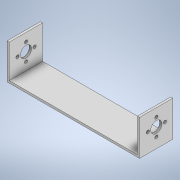
# Autodesk Inventor part: Rotate Brace
Saved by Autodesk Inventor 2020 (Build 240168000, 168)
## iProperties
Created: 2020-01-19
Part Number: Rotate Brace
Material: Generic
Document SubType Name: Modeling
Designer: tdmp4
Density: 1 g/cm^3
Appearance: Default
Author: tdmp4
Autodesk Inventor part; units mm, degrees
ref_plane "YZ Plane" through (0, 0, 0) normal (1, 0, 0) x (0, 1, 0)
ref_plane "XZ Plane" through (0, 0, 0) normal (0, 1, 0) x (-1, 0, 0)
ref_plane "XY Plane" through (0, 0, 0) normal (0, 0, 1) x (1, 0, 0)
sketch "Sketch1" plane through (0, 0, 0) normal (0, 1, 0) x (-1, 0, 0)
  line L0 (0, 0) -> (151.4602, 0)
  line L1 (151.4602, 0) -> (151.4602, -38.1)
  line L2 (151.4602, -38.1) -> (0, -38.1)
  line L3 (0, -38.1) -> (0, 0)
  dimension "d0" = 151.4602
  dimension "d1" = 38.1
  constraints: 8 end point, 2 parallel, 1 horizontal, 1 perpendicular
  measures "d0" distance of L1.end L2.end
  measures "d1" distance of L2.end L0.start
extrude "Extrusion1" add sketch "Sketch1" along normal blind 2.54
sketch "Sketch3" plane through (0, 0, 0) normal (1, 0, 0) x (0, 0, -1)
  circle A0 centre (19.05, 31.369) radius 1.7907
  circle A1 centre (28.829, 21.59) radius 1.7907
  circle A2 centre (19.05, 11.811) radius 1.7907
  circle A3 centre (9.271, 21.59) radius 1.7907
  circle A4 centre (19.05, 21.59) radius 6.35
  point P0 (0, 0)
  dimension "d12" = 12.7
  constraints: 5 centre point
  measures "d12" diameter of A4
sketch "Sketch4" plane through (0, 2.54, 0) normal (0, 1, 0) x (1, 0, 0)
  line L0 (0, 38.1) -> (-151.4602, 38.1) projected
  line L1 (0, 0) -> (-2.451, 0)
  line L2 (-2.451, 0) -> (-2.451, 38.1)
  line L3 (-2.451, 38.1) -> (0, 38.1)
  line L4 (0, 38.1) -> (0, 0)
  line L5 (-151.4602, 38.1) -> (-151.4602, 0) projected
  line L6 (-151.4602, 0) -> (-148.9202, 0)
  line L7 (-148.9202, 0) -> (-148.9202, 38.1)
  line L8 (-148.9202, 38.1) -> (-151.4602, 38.1)
  line L9 (-151.4602, 38.1) -> (-151.4602, 0)
  point P0 (0, 38.1)
  point P1 (-148.9202, 38.1)
  dimension "d17" = 2.54
  constraints: 16 end point, 4 parallel, 2 horizontal, 2 perpendicular, 2 point on line
  measures "d17" distance of L5.end L6.end
extrude "Extrusion3" add sketch "Sketch4" along normal blind 38.1
extrude "Extrusion4" cut sketch "Sketch3" against normal blind 203.2
body "Solid1"
